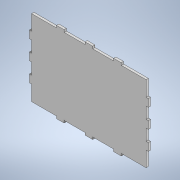
# Autodesk Inventor part: Врех и низ
Saved by Autodesk Inventor 2021 (Build 250183000, 183)
## iProperties
Created: 2021-04-11
Part Number: Врех и низ
Material: Типовые
Document SubType Name: Modeling
Designer: user
Density: 1 g/cm^3
Appearance: По умолчанию
Author: user
Autodesk Inventor part; units mm, degrees
ref_plane "YZ Plane" through (0, 0, 0) normal (1, 0, 0) x (0, 1, 0)
ref_plane "XZ Plane" through (0, 0, 0) normal (0, 1, 0) x (-1, 0, 0)
ref_plane "XY Plane" through (0, 0, 0) normal (0, 0, 1) x (1, 0, 0)
sketch "Эскиз1" plane through (0, 0, 0) normal (0, 0, 1) x (1, 0, 0)
  line L0 (0, 53) -> (5, 53)
  line L1 (5, 53) -> (5, 50)
  line L2 (32.5, 53) -> (42.5, 53)
  line L3 (42.5, 53) -> (42.5, 50)
  line L4 (32.5, 50) -> (32.5, 53)
  line L5 (78, 30) -> (75, 30)
  line L6 (75, 20) -> (78, 20)
  line L7 (78, 20) -> (78, 30)
  line L8 (78, 5) -> (75, 5)
  line L9 (78, 0) -> (78, 5)
  line L10 (5, 50) -> (32.5, 50)
  line L11 (42.5, 50) -> (75, 50)
  line L12 (5, 50) -> (32.5, 50)
  line L13 (42.5, 50) -> (75, 50)
  line L14 (75, 50) -> (75, 30)
  line L15 (75, 20) -> (75, 5)
  line L16 (75, 50) -> (75, 30)
  line L17 (75, 20) -> (75, 5)
  line L18 (32.5, -53) -> (42.5, -53)
  line L19 (32.5, -50) -> (32.5, -53)
  line L20 (5, -50) -> (32.5, -50)
  line L21 (5, -50) -> (32.5, -50)
  line L22 (5, -53) -> (5, -50)
  line L23 (0, -53) -> (5, -53)
  line L24 (42.5, -53) -> (42.5, -50)
  line L25 (42.5, -50) -> (75, -50)
  line L26 (42.5, -50) -> (75, -50)
  line L27 (75, -50) -> (75, -30)
  line L28 (75, -50) -> (75, -30)
  line L29 (78, -30) -> (75, -30)
  line L30 (75, -20) -> (78, -20)
  line L31 (78, -20) -> (78, -30)
  line L32 (75, -20) -> (75, -5)
  line L33 (75, -20) -> (75, -5)
  line L34 (78, -5) -> (75, -5)
  line L35 (78, 0) -> (78, -5)
  line L36 (-32.5, 53) -> (-42.5, 53)
  line L37 (-32.5, 50) -> (-32.5, 53)
  line L38 (-5, 50) -> (-32.5, 50)
  line L39 (-5, 50) -> (-32.5, 50)
  line L40 (-5, 53) -> (-5, 50)
  line L41 (0, 53) -> (-5, 53)
  line L42 (-42.5, 53) -> (-42.5, 50)
  line L43 (-42.5, 50) -> (-75, 50)
  line L44 (-75, 50) -> (-75, 30)
  line L45 (-75, 50) -> (-75, 30)
  line L46 (-78, 30) -> (-75, 30)
  line L47 (-75, 20) -> (-78, 20)
  line L48 (-78, 20) -> (-78, 30)
  line L49 (-75, 20) -> (-75, 5)
  line L50 (-75, 20) -> (-75, 5)
  line L51 (-42.5, 50) -> (-75, 50)
  line L52 (-32.5, -53) -> (-42.5, -53)
  line L53 (-32.5, -50) -> (-32.5, -53)
  line L54 (-5, -50) -> (-32.5, -50)
  line L55 (-5, -50) -> (-32.5, -50)
  line L56 (0, -53) -> (-5, -53)
  line L57 (-5, -53) -> (-5, -50)
  line L58 (-78, 5) -> (-75, 5)
  line L59 (-78, 0) -> (-78, 5)
  line L60 (-78, 0) -> (-78, -5)
  line L61 (-78, -5) -> (-75, -5)
  line L62 (-75, -20) -> (-75, -5)
  line L63 (-75, -20) -> (-75, -5)
  line L64 (-75, -20) -> (-78, -20)
  line L65 (-78, -30) -> (-75, -30)
  line L66 (-78, -20) -> (-78, -30)
  line L67 (-75, -50) -> (-75, -30)
  line L68 (-75, -50) -> (-75, -30)
  line L69 (-42.5, -50) -> (-75, -50)
  line L70 (-42.5, -50) -> (-75, -50)
  line L71 (-42.5, -53) -> (-42.5, -50)
  point P0 (37.5, 50)
  point P1 (75, 25)
  point P2 (37.5, -50)
  point P3 (75, -25)
  point P4 (-37.5, 50)
  point P5 (-37.5, -50)
  constraints: 144 end point, 6 horizontal, 6 perpendicular, 4 collinear, 2 parallel
extrude "Выдавливание1" add sketch "Эскиз1" along normal blind 3
